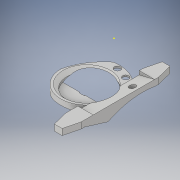
# Autodesk Inventor part: headppost_Turi_2gen
Saved by Autodesk Inventor 2018 (Build 220112000, 112)
## iProperties
Created: 2017-08-21
Part Number: headppost_Turi_2gen
Material: Generic
Document SubType Name: Modeling
Designer: Gergely Turi
Density: 1 g/cm^3
Appearance: Default
Author: Gergely Turi
Autodesk Inventor part; units mm, degrees
ref_plane "YZ Plane" through (0, 0, 0) normal (1, 0, 0) x (0, 1, 0)
ref_plane "XZ Plane" through (0, 0, 0) normal (0, 1, 0) x (-1, 0, 0)
ref_plane "XY Plane" through (0, 0, 0) normal (0, 0, 1) x (1, 0, 0)
sketch "Sketch1" plane through (0, 0, 0) normal (1, 0, 0) x (0, 1, 0)
  line L0 (0, 0) -> (1.27, 0)
  line L1 (1.27, 0) -> (1.27, 22.3012)
  line L2 (1.27, 22.3012) -> (0, 22.3012)
  arc A0 (0, 3.7418) -> (-1.4817, 13.594) centre (-15.6464, 6.4262) ccw
  line L3 (0, 18.4404) -> (-1.4817, 13.594)
  line L4 (0, 22.3012) -> (0, 18.4404)
  line L5 (0, 3.7418) -> (0, 0)
  dimension "d0" = 1.27
  dimension "d1" = 22.3012
  dimension "d2" = 31.75
  dimension "d3" = 6.4262
  dimension "d4" = 16.9164
  dimension "d6" = 3.8608
  constraints: 12 end point, 3 parallel, 2 point on circle, 1 centre point, 1 horizontal, 1 perpendicular
  measures "d0" distance of L2.end L1.end
  measures "d1" distance of L1.end L0.end
  measures "d2" diameter of A0
  measures "d3" distance from line of L0 A0.centre
  measures "d4" distance from line of L1 A0.centre
  measures "d6" distance of L3.start L2.end
extrude "Extrusion1" add sketch "Sketch1" along normal blind 12.3444
sketch "Sketch2" plane through (0, 1.27, 22.3012) normal (0, 1, 0) x (1, 0, 0)
  line L0 (0, 0) -> (12.3444, 0) projected
  line L1 (9.9568, 0) -> (9.1694, 3.1581)
  line L2 (11.557, 0) -> (12.3444, 3.1581)
  line L3 (9.1694, 3.1581) -> (9.1694, 19.1431)
  line L4 (12.3444, 22.3012) -> (12.3444, 0) projected
  line L5 (10.7569, 0) -> (10.7569, 22.3012)
  line L6 (0, 22.3012) -> (12.3444, 22.3012) projected
  line L7 (9.9568, 22.3012) -> (9.1694, 19.1431)
  line L8 (11.557, 22.3012) -> (12.3444, 19.1431)
  line L9 (9.1694, 19.1431) -> (0, 19.1431)
  line L10 (9.1694, 3.1581) -> (0, 3.1581)
  line L11 (0, 22.3012) -> (0, 0) projected
  line L12 (0, 19.1431) -> (0, 22.3012)
  line L13 (0, 22.3012) -> (9.9568, 22.3012)
  line L14 (0, 3.1581) -> (0, 0)
  dimension "d9" = 1.6002
  dimension "d13" = 28
  dimension "d14" = 3.175
  dimension "d15" = 1.5875
  dimension "d16" = 1.6002
  dimension "d17" = 28
  constraints: 22 end point, 7 point on line, 3 collinear, 2 horizontal, 2 vertical, 2 other
  measures "d9" distance of L1.start L2.start
  measures "d13" angle of L1 L2
  measures "d14" distance between parallel lines of L4 L3
  measures "d15" distance between parallel lines of L3 L5
  measures "d16" distance of L8.start L7.start
  measures "d17" angle of L8 L7
extrude "Extrusion2" cut sketch "Sketch2" against normal blind 25.4 contours L11 L10 L1 L0 | L11 L6 L7 L9 | L2 L4 L0 | L6 L4 L8
sketch "Sketch8" plane through (0, 1.27, 3.1581) normal (0, 1, 0) x (1, 0, 0)
  line L0 (9.1694, -0.8043) -> (0, -0.8043)
  line L1 (9.1694, 0) -> (0, 0) projected
  line L2 (0, -0.8043) -> (9.1694, -0.8043)
  line L3 (9.1694, -0.8043) -> (9.1694, 0)
  line L4 (9.1694, 0) -> (0, 0)
  line L5 (0, 0) -> (0, -0.8043)
  point P0 (0, 3.1581)
  point P1 (0, -10.4309)
  constraints: 10 end point, 2 parallel, 1 horizontal, 1 perpendicular
extrude "Extrusion5" cut sketch "Sketch8" against normal blind 25.4
sketch "Sketch9" plane through (9.9568, 1.27, 22.3012) normal (0, 1, 0) x (1, 0, 0)
  line L0 (-10.6834, 14.9326) -> (-5.2324, 18.3388)
  line L1 (-5.2324, 18.3388) -> (-10.6834, 18.3388)
  line L2 (-10.6834, 18.3388) -> (-10.6834, 14.9326)
  line L3 (-0.7874, 19.1431) -> (-0.7874, 18.3388) projected
  line L4 (-0.7874, 18.3388) -> (-9.9568, 18.3388) projected
  point P0 (-9.9568, 22.3012)
  dimension "d41" = 32
  dimension "d42" = 4.445
  constraints: 6 end point, 1 collinear, 1 horizontal, 1 perpendicular
  measures "d41" angle of L1 L0
  measures "d42" distance from line of L3 L0.end
extrude "Extrusion6" cut sketch "Sketch9" against normal blind 25.4
sketch "Sketch14" plane through (9.9568, 1.27, 22.3012) normal (0, 1, 0) x (1, 0, 0)
  circle A0 centre (-4.5896, 11.2866) radius 1.143
  line L0 (-5.2273, 9.7597) -> (-3.813, 11.1739)
  line L1 (-5.2273, 9.7597) -> (-3.2273, 9.7597) construction
  line L2 (-3.813, 11.1739) -> (-5.2273, 11.1739)
  line L3 (-5.2273, 11.1739) -> (-5.2273, 9.7597)
  line L4 (-3.813, 11.1739) -> (-3.813, 9.7597)
  line L5 (-3.813, 9.7597) -> (-5.2273, 9.7597)
  circle A1 centre (-4.5201, 10.4668) radius 3.175
  point P0 (-9.9568, 22.3012)
  dimension "d78" = 2.286
  dimension "d86" = 2
  dimension "d87" = 45
  dimension "d88" = 6.35
  constraints: 12 end point, 2 centre point, 1 equal length, 1 horizontal, 1 midpoint, 1 perpendicular, 1 symmetric about line
  measures "d78" diameter of A0
  measures "d86" distance of L0.start L0.end
  measures "d87" angle of L1 L0
  measures "d88" diameter of A1
extrude "Extrusion11" cut sketch "Sketch14" against normal blind 25.4 contours A0 L4 L2 L3 | L3 L2 L0 A0 | A0 L0 L4
sketch "Sketch15" plane through (9.9568, 1.27, 22.3012) normal (0, 1, 0) x (1, 0, 0)
  circle A0 centre (-4.5896, 11.2866) radius 1.143 projected
  circle A1 centre (-4.5896, 11.2866) radius 0.9525
  circle A2 centre (-4.5896, 11.2866) radius 4.1275
  point P0 (-9.9568, 22.3012)
  dimension "d82" = 1.905
  dimension "d83" = 8.255
  constraints: 2 centre point, 2 coincident
  measures "d82" diameter of A1
  measures "d83" diameter of A2
extrude "Extrusion12" cut sketch "Sketch15" against normal blind 2.032 contours A2
sketch "Sketch19" plane through (9.9568, 1.27, 22.3012) normal (0, 1, 0) x (1, 0, 0)
  circle A0 centre (1.0564, 15.0967) radius 0.635
  circle A1 centre (-1.7204, 16.4692) radius 0.635
  circle A2 centre (-4.1782, 17.2168) radius 0.635
  point P0 (-9.9568, 22.3012)
  dimension "d102" = 1.27
  dimension "d103" = 1.27
  dimension "d104" = 1.27
  constraints: 3 centre point
  measures "d102" diameter of A0
  measures "d103" diameter of A1
  measures "d104" diameter of A2
extrude "Extrusion17" cut sketch "Sketch19" against normal blind 2.286
sketch "Sketch27" plane through (9.1694, 0.0362, 3.9624) normal (0, 0, -1) x (-1, 0, 0)
  line L0 (0, 1.2338) -> (0, -0.0362) projected
  line L1 (9.1694, 1.2338) -> (9.1694, 0.1848) projected
  line L2 (0, 1.2338) -> (9.1694, 1.2338)
  line L3 (9.1694, 1.2338) -> (9.1694, 0.4718)
  line L4 (9.1694, 0.4718) -> (0, 0.4718)
  line L5 (0, 0.4718) -> (0, 1.2338)
  point P0 (9.1694, -0.0362)
  dimension "d122" = 0.762
  constraints: 8 end point, 2 parallel, 1 horizontal, 1 perpendicular, 1 point on line
  measures "d122" distance of L2.end L3.end
extrude "Extrusion22" cut sketch "Sketch27" against normal through all
sketch "Sketch29" plane through (4.7244, 0.508, 3.9624) normal (0, 1, 0) x (1, 0, 0)
  arc A0 (-0.0195, -7.9838) -> (1.3051, -7.9838) centre (0.6428, -7.0522) ccw projected
  arc A1 (-4.7244, -7.0522) -> (4.445, -10.8404) centre (0.6428, -7.0522) ccw
  line L0 (-4.7244, -15.1807) -> (-4.7244, -2.9521) projected
  line L1 (4.445, -8.6583) -> (4.445, -15.1807) projected
  line L2 (4.445, -10.8404) -> (4.445, -15.1807)
  line L3 (4.445, -15.1807) -> (-4.7244, -15.1807)
  point P0 (-4.7244, 3.9624)
  constraints: 4 end point, 2 point on circle, 2 point on line, 1 centre point, 1 coincident, 1 collinear, 1 perpendicular, 1 tangent
extrude "Extrusion23" cut sketch "Sketch29" against normal through all
sketch "Sketch30" plane through (4.7244, 0.508, 3.9624) normal (0, 1, 0) x (1, 0, 0)
  line L0 (0, 0) -> (-4.7244, -2.9521) projected
  line L1 (-4.7244, -2.9521) -> (-4.7244, -7.0522) projected
  arc A0 (0, 0) -> (-4.7244, -7.0522) centre (6.8812, -9.7184) ccw
  line L2 (-4.7244, -7.0522) -> (-4.7244, -2.9521)
  point P0 (-4.7244, 3.9624)
  constraints: 2 end point, 2 point on circle, 1 centre point, 1 collinear
extrude "Extrusion24" cut sketch "Sketch30" against normal through all
sketch "Sketch32" plane through (9.1694, 0.0362, 3.9624) normal (0, 0, -1) x (-1, 0, 0)
  line L0 (4.445, 0.4718) -> (0, 0.4718) projected
  line L1 (0, 0.4718) -> (0, 1.2338)
  line L2 (0, 1.2338) -> (-3.175, 1.2338)
  line L3 (0, 0.4718) -> (0, 0) projected
  line L4 (-3.175, 1.2338) -> (0, 0.4718)
  point P0 (9.1694, -0.0362)
  constraints: 6 end point, 1 perpendicular, 1 vertical
extrude "Extrusion26" cut sketch "Sketch32" against normal blind 12.7
sketch "Sketch37" plane through (4.7244, 0.508, 3.9624) normal (0, 1, 0) x (1, 0, 0)
  arc A0 (4.445, -5.4461) -> (4.445, -8.6583) centre (0.6428, -7.0522) ccw projected
  arc A1 (4.445, -1.4721) -> (-0.5374, -0.4038) centre (0.6428, -7.0522) ccw
  line L0 (4.445, 0) -> (4.445, -5.4461) projected
  line L1 (4.445, -1.4721) -> (4.445, 0)
  line L2 (4.445, 0) -> (0, 0)
  arc A2 (0, 0) -> (-4.7244, -7.0522) centre (6.8812, -9.7184) ccw projected
  line L3 (0, 0) -> (4.445, 0) projected
  arc A3 (0, 0) -> (-0.5374, -0.4038) centre (1.2434, -2.2145) ccw
  point P0 (-4.7244, 3.9624)
  constraints: 5 point on circle, 4 end point, 2 centre point, 1 coincident, 1 collinear, 1 perpendicular, 1 point on line
extrude "Extrusion27" cut sketch "Sketch37" against normal blind 12.7 contours A1 A2 L2 L0
chamfer "Chamfer4" distance 0.762 angle 45 1 edges at (1.2397, 0.508, 11.0146)
sketch "Sketch38" plane through (9.9568, -0.762, 22.3012) normal (0, 1, 0) x (1, 0, 0)
  ellipse E0 centre (-3.5768, 11.2866) end of major axis (-7.7968, 11.2866) minor radius 4.0967 (-3.9624, 7.207) -> (-0.7874, 8.2124) ccw projected
  arc A0 (-4.2943, 7.198) -> (-4.2943, 15.3752) centre (-3.5768, 11.2866) ccw
  arc A1 (-3.9624, 7.207) -> (-2.158, 14.6218) centre (-4.5896, 11.2866) ccw projected
  arc A2 (-4.2943, 7.198) -> (-4.2943, 15.3752) centre (-4.5896, 11.2866) ccw
  point P0 (-9.9568, 22.3012)
  constraints: 4 point on circle, 2 centre point, 2 coincident, 1 other
extrude "Extrusion28" cut sketch "Sketch38" along normal blind 12.7
sketch "Sketch39" plane through (5.3672, 0.508, 11.0146) normal (0, 1, 0) x (1, 0, 0)
  point P0 (-5.3672, 11.0146)
equation "\"d15\" = 0.5 * d14"
body "Solid1"
